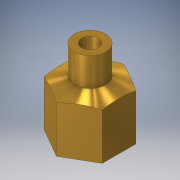
# Autodesk Inventor part: am-2381
Saved by Autodesk Inventor 2016 SP2 (Build 200236200, 236)
## iProperties
Created: 2017-03-28
Part Number: am-2381
Material: Brass
Document SubType Name: Modeling
Designer: smiku
Mass: 31.8591 g
Surface Area: 27.2455 cm^2
Volume: 3.75255 cm^3
Density: 8.49 g/cm^3
Appearance: Brass - Polished
Author: smiku
Autodesk Inventor part; units mm, degrees
ref_plane "YZ Plane" through (0, 0, 0) normal (1, 0, 0) x (0, 1, 0)
ref_plane "XZ Plane" through (0, 0, 0) normal (0, 1, 0) x (-1, 0, 0)
sketch "Sketch1" plane through (0, 0, 0) normal (0, 1, 0) x (-1, 0, 0)
  circle A0 centre (0, 0) radius 9.5504 construction
  line L0 (9.5504, -5.5139) -> (0, -11.0279)
  line L1 (0, -11.0279) -> (-9.5504, -5.5139)
  line L2 (-9.5504, -5.5139) -> (-9.5504, 5.5139)
  line L3 (-9.5504, 5.5139) -> (0, 11.0279)
  line L4 (0, 11.0279) -> (9.5504, 5.5139)
  line L5 (9.5504, 5.5139) -> (9.5504, -5.5139)
  circle A1 centre (0, 0) radius 6.35
  point P0 (9.5504, 0)
  dimension "d0" = 19.1008
  dimension "d1" = 12.7
  constraints: 12 end point, 3 coincident, 1 centre point, 1 horizontal alignment, 1 midpoint, 1 vertical, 15 other
  measures "d1" diameter of A1
extrude "Extrusion1" add sketch "Sketch1" along normal blind 15.24
ref_plane "Work Plane1" through (0, 26.8224, 0) normal (0, -1, 0) x (1, 0, 0)
sketch "Sketch2" plane through (0, 26.8224, 0) normal (0, -1, 0) x (1, 0, 0)
  circle A0 centre (0, 0) radius 2.7559
  circle A1 centre (0, 0) radius 5.1562
  dimension "d5" = 5.5118
  dimension "d6" = 10.3124
  constraints: 2 centre point, 2 coincident
  measures "d5" diameter of A0
  measures "d6" diameter of A1
extrude "Extrusion2" add sketch "Sketch2" along normal blind 9.3726
sketch "Sketch3" plane through (0, 0, 0) normal (1, 0, 0) x (0, 1, 0)
  line L0 (15.24, -11.0279) -> (0, -11.0279) construction
  line L1 (0, -11.0279) -> (0, -6.35) construction
  line L2 (0, -6.35) -> (15.24, -6.35) construction
  line L3 (15.24, -6.35) -> (15.24, -11.0279) construction
  line L4 (0, 11.0279) -> (15.24, 11.0279) construction
  line L5 (15.24, 11.0279) -> (15.24, 6.35) construction
  line L6 (15.24, 6.35) -> (0, 6.35) construction
  line L7 (0, 6.35) -> (0, 11.0279) construction
  line L8 (26.8224, -5.1562) -> (17.4498, -5.1562) construction
  line L9 (17.4498, -5.1562) -> (17.4498, -2.7559) construction
  line L10 (17.4498, -2.7559) -> (26.8224, -2.7559) construction
  line L11 (26.8224, -2.7559) -> (26.8224, -5.1562) construction
  line L12 (17.4498, 5.1562) -> (26.8224, 5.1562) construction
  line L13 (26.8224, 5.1562) -> (26.8224, 2.7559) construction
  line L14 (26.8224, 2.7559) -> (17.4498, 2.7559) construction
  line L15 (17.4498, 2.7559) -> (17.4498, 5.1562) construction
  line L16 (17.4498, 5.1562) -> (17.4498, -5.1562) projected
  line L17 (17.4498, -2.7559) -> (17.4498, -5.1562)
  line L18 (17.4498, -5.1562) -> (15.24, -11.0279)
  line L19 (15.24, -6.35) -> (17.4498, -2.7559)
  line L20 (0, 0) -> (26.8224, 0) construction
  line L21 (15.24, -6.35) -> (15.24, -11.0279)
  constraints: 10 end point, 2 vertical, 1 horizontal
revolve "Revolution1" add sketch "Sketch3" angle 360 about axis through (0, 0, 0) along (0, 1, 0)
sketch "Sketch4" plane through (0, 0, 0) normal (0, -1, 0) x (1, 0, 0)
  circle A0 centre (0, 0) radius 6.35 construction
  line L0 (9.5504, -5.5139) -> (0, -11.0279) projected
  line L1 (0, -11.0279) -> (-9.5504, -5.5139) projected
  line L2 (-9.5504, -5.5139) -> (-9.5504, 5.5139) projected
  line L3 (-9.5504, 5.5139) -> (0, 11.0279) projected
  line L4 (0, 11.0279) -> (9.5504, 5.5139) projected
  line L5 (9.5504, 5.5139) -> (9.5504, -5.5139) projected
  line L6 (9.5504, 5.5139) -> (0, 11.0279) projected
  circle A1 centre (0, 0) radius 11.0279
  constraints: 1 coincident, 1 vertical alignment, 2 other
extrude "Extrusion3" cut sketch "Sketch4" against normal through all contours A1 L0 | L5 A1 | A1 L1 | L4 A1 | A1 L2 | L3 A1
body "Solid1"
